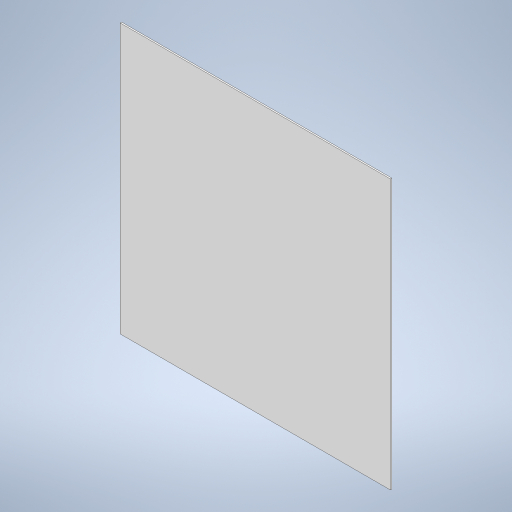
# Autodesk Inventor part: plate_front
Saved by Autodesk Inventor 2023 (Build 270158000, 158)
## iProperties
Created: 2023-08-22
Part Number: plate_front
Material: Polystyrene
Document SubType Name: Modeling
Designer: chriboehm
Density: 1.021 g/cm^3
Appearance: White
Author: chriboehm
Autodesk Inventor part; units mm, degrees
ref_plane "YZ Plane" through (0, 0, 0) normal (1, 0, 0) x (0, 1, 0)
ref_plane "XZ Plane" through (0, 0, 0) normal (0, 1, 0) x (-1, 0, 0)
ref_plane "XY Plane" through (0, 0, 0) normal (0, 0, 1) x (1, 0, 0)
sketch "Sketch1" plane through (0, 0, 0) normal (0, 0, 1) x (1, 0, 0)
  line L0 (0, 0) -> (542, 0)
  line L1 (542, 0) -> (542, 540)
  line L2 (542, 540) -> (0, 540)
  line L3 (0, 540) -> (0, 0)
  dimension "d0" = 542
  dimension "d1" = 540
  constraints: 8 end point, 2 parallel, 1 horizontal, 1 perpendicular
  measures "d0" distance of L1.end L2.end
  measures "d1" distance between parallel lines of L0 L2
extrude "Extrusion1" add sketch "Sketch1" along normal blind 3
body "Solid1"
